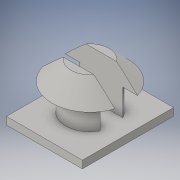
# Autodesk Inventor part: Snap
Saved by Autodesk Inventor 2016 (Build 200138000, 138)
## iProperties
Created: 2016-10-07
Part Number: Snap
Material: Generic
Document SubType Name: Modeling
Designer: lachesis
Density: 1 g/cm^3
Appearance: Default
Author: lachesis
Autodesk Inventor part; units mm, degrees
ref_plane "YZ Plane" through (0, 0, 0) normal (1, 0, 0) x (0, 1, 0)
ref_plane "XZ Plane" through (0, 0, 0) normal (0, 1, 0) x (-1, 0, 0)
ref_plane "XY Plane" through (0, 0, 0) normal (0, 0, 1) x (1, 0, 0)
sketch "Sketch1" plane through (0, 0, 0) normal (0, 0, 1) x (1, 0, 0)
  line L0 (0, 5) -> (0, 0)
  line L1 (0, 0) -> (5, 0)
  line L2 (5, 0) -> (0, 5)
  dimension "d45" = 5
  dimension "d46" = 5
  constraints: 6 end point, 1 coincident, 1 perpendicular, 1 vertical
  measures "d45" distance of L0.start L0.end
  measures "d46" distance of L0.end L1.end
revolve "Revolution1" add sketch "Sketch1" angle 360 about axis through (0, 5, 0) along (0, -1, 0)
sketch "Sketch2" plane through (0, 0, 0) normal (0, -1, 0) x (1, 0, 0)
  circle A0 centre (0, 0) radius 3.2
  dimension "d3" = 6.4
  constraints: 1 centre point, 1 coincident
  measures "d3" diameter of A0
extrude "Extrusion1" add sketch "Sketch2" along normal blind 3.5
sketch "Sketch3" plane through (0, -3.5, 0) normal (0, -1, 0) x (1, 0, 0)
  circle A0 centre (0, 0) radius 5 projected
  line L0 (-5.5, 1.5) -> (5.5, 1.5)
  line L1 (5.5, 1.5) -> (5.5, -1.5)
  line L2 (5.5, -1.5) -> (-5.5, -1.5)
  line L3 (-5.5, -1.5) -> (-5.5, 1.5)
  point P0 (0, 1.5)
  point P1 (5.5, 0)
  dimension "d27" = 0.5
  dimension "d28" = 3
  constraints: 8 end point, 2 midpoint, 2 parallel, 1 horizontal, 1 horizontal alignment, 1 perpendicular, 1 vertical alignment
  measures "d27" distance edge to line of A0 L1
  measures "d28" distance between parallel lines of L2 L0
extrude "Extrusion2" cut sketch "Sketch3" against normal through all contours A0 L2 L0 | A0 L0 L1 L2 | A0 L2 L3 L0
sketch "Sketch4" plane through (0, -3.5, 0) normal (0, -1, 0) x (1, 0, 0)
  line L0 (4.9945, 6) -> (-4.9945, 6)
  line L1 (-4.9945, 6) -> (-4.9945, -6)
  line L2 (-4.9945, -6) -> (4.9945, -6)
  line L3 (4.9945, -6) -> (4.9945, 6)
  arc A0 (-1.5, 3.7021) -> (-1.5, -3.7021) centre (0, 0) ccw projected
  arc A1 (-1.5, 3.4857) -> (-1.5, -3.4857) centre (0, 0) ccw projected
  line L4 (-1.5, 3.4857) -> (-1.5, 3.7021) projected
  line L5 (-1.5, -3.7021) -> (-1.5, -3.4857) projected
  arc A2 (4.7697, 1.5) -> (-4.7697, 1.5) centre (0, 0) ccw projected
  point P0 (4.9945, 0)
  point P1 (0, -6)
  dimension "d18" = 1
  dimension "d42" = 1
  constraints: 8 end point, 2 midpoint, 2 parallel, 1 horizontal, 1 horizontal alignment, 1 perpendicular, 1 vertical alignment
  measures "d18" distance edge to line of A0 L1
  measures "d42" distance edge to line of A2 L0
extrude "Extrusion3" add sketch "Sketch4" along normal blind 1 contours L3 L2 L1 L0 | L4 A1 L5 A0
sketch "Sketch9" plane through (4.9945, -3.5, 6) normal (1, 0, 0) x (0, 0, -1)
  line L0 (3.5, 7) -> (8.5, 7)
  line L1 (8.5, 7) -> (8.5, 6)
  line L2 (8.5, 6) -> (3.5, 6)
  line L3 (3.5, 6) -> (3.5, 7)
  line L4 (4.5, 7) -> (1, 3.5) projected
  line L5 (4.9945, 3.5) -> (4.9945, 7) projected
  line L6 (7.5, 7) -> (11, 3.5) projected
  point P0 (6, 3.5)
  point P1 (4.5, 3.5)
  point P2 (7.5, 3.5)
  point P3 (4.9945, 3.5)
  point P4 (11, 3.5)
  dimension "d47" = 1
  constraints: 8 end point, 2 parallel, 2 point on line, 1 horizontal, 1 perpendicular, 3 other
  measures "d47" distance between parallel lines of L2 L0
extrude "Extrusion8" cut sketch "Sketch9" against normal through all
equation "\"d46\" = d45"
equation "\"d27\" = d22"
equation "\"d28\" = d19"
equation "\"d42\" = d18"
equation "\"d22\" = 0.5"
equation "\"d19\" = 3"
body "Solid1"
